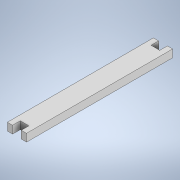
# Autodesk Inventor part: FondV2
Saved by Autodesk Inventor 2020 (Build 240168000, 168)
## iProperties
Created: 2019-11-14
Part Number: FondV2
Material: Générique
Document SubType Name: Modeling
Designer: erwan
Density: 1 g/cm^3
Appearance: Par défaut
Author: erwan
Autodesk Inventor part; units mm, degrees
ref_plane "YZ Plane" through (0, 0, 0) normal (1, 0, 0) x (0, 1, 0)
ref_plane "XZ Plane" through (0, 0, 0) normal (0, 1, 0) x (-1, 0, 0)
ref_plane "XY Plane" through (0, 0, 0) normal (0, 0, 1) x (1, 0, 0)
sketch "Esquisse1" plane through (0, 0, 0) normal (0, 1, 0) x (-1, 0, 0)
  line L0 (0, 0) -> (-15, 0)
  line L1 (-55, 0) -> (-55, -419)
  line L2 (-55, -419) -> (-40, -419)
  line L3 (0, -419) -> (0, 0)
  line L4 (-40, -419) -> (-40, -397)
  line L5 (-40, -397) -> (-15, -397)
  line L6 (-15, -397) -> (-15, -419)
  line L7 (-15, -419) -> (0, -419)
  line L8 (-40, 0) -> (-40, -22)
  line L9 (-40, -22) -> (-15, -22)
  line L10 (-15, -22) -> (-15, 0)
  line L11 (-40, 0) -> (-55, 0)
  dimension "d0" = 419
  dimension "d1" = 55
  dimension "d2" = 22
  dimension "d3" = 25
  dimension "d4" = 15
  dimension "d5" = 15
  dimension "d6" = 22
  dimension "d7" = 25
  dimension "d8" = 15
  dimension "d9" = 15
  constraints: 24 end point, 7 parallel, 2 horizontal, 2 perpendicular
  measures "d0" distance between parallel lines of L0 L2
  measures "d1" distance between parallel lines of L1 L3
  measures "d2" distance between parallel lines of L5 L2
  measures "d3" distance between parallel lines of L4 L6
  measures "d4" distance between parallel lines of L6 L3
  measures "d5" distance between parallel lines of L1 L4
  measures "d6" distance between parallel lines of L0 L9
  measures "d7" distance between parallel lines of L8 L10
  measures "d8" distance between parallel lines of L3 L10
  measures "d9" distance between parallel lines of L8 L1
extrude "Extrusion1" add sketch "Esquisse1" along normal blind 22
